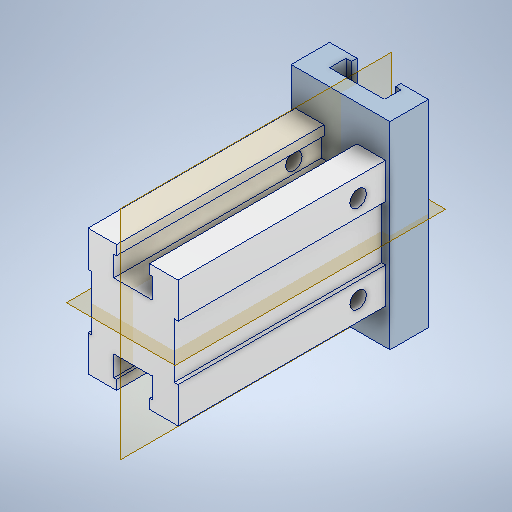
# Autodesk Inventor part: Cylinder
Saved by Autodesk Inventor 2025 (Build 290162000, 162)
## iProperties
Created: 2024-09-26
Part Number: Cylinder
Material: Aluminum 6061
Document SubType Name: Modeling
Designer: DMIADX
Density: 2.7 g/cm^3
Appearance: Aluminum - Flat
Author: DMIADX
Autodesk Inventor part; units mm, degrees
ref_plane "XY Plane" through (0, 0, 0) normal (0, 0, 1) x (1, 0, 0)
sketch "Sketch1" plane through (0, 0, 0) normal (0, 0, 1) x (1, 0, 0)
  line L0 (8.2, -11.5) -> (-8.2, -11.5)
  line L1 (-8.2, -11.5) -> (-8.2, 11.5)
  line L2 (-8.2, 11.5) -> (8.2, 11.5)
  line L3 (8.2, 11.5) -> (8.2, -11.5)
  line L4 (8.2, -11.5) -> (-8.2, 11.5) construction
  line L5 (-8.2, -11.5) -> (8.2, 11.5) construction
  line L6 (8.2, -5) -> (-8.2, -5)
  line L7 (-8.2, -5) -> (-8.2, 5)
  line L8 (-8.2, 5) -> (8.2, 5)
  line L9 (8.2, 5) -> (8.2, -5)
  line L10 (8.2, -5) -> (-8.2, 5) construction
  line L11 (-8.2, -5) -> (8.2, 5) construction
  line L12 (7.5, -5) -> (-7.5, -5)
  line L13 (-7.5, -5) -> (-7.5, 5)
  line L14 (-7.5, 5) -> (7.5, 5)
  line L15 (7.5, 5) -> (7.5, -5)
  line L16 (7.5, -5) -> (-7.5, 5) construction
  line L17 (-7.5, -5) -> (7.5, 5) construction
  line L18 (3, -11.5) -> (-3, -11.5)
  line L19 (-3, -11.5) -> (-3, 11.5)
  line L20 (-3, 11.5) -> (3, 11.5)
  line L21 (3, 11.5) -> (3, -11.5)
  line L22 (3, -11.5) -> (-3, 11.5) construction
  line L23 (-3, -11.5) -> (3, 11.5) construction
  line L24 (3.5, -9.75) -> (-3.5, -9.75)
  line L25 (-3.5, -9.75) -> (-3.5, 9.75)
  line L26 (-3.5, 9.75) -> (3.5, 9.75)
  line L27 (3.5, 9.75) -> (3.5, -9.75)
  line L28 (3.5, -9.75) -> (-3.5, 9.75) construction
  line L29 (-3.5, -9.75) -> (3.5, 9.75) construction
  line L30 (3.5, -6) -> (-3.5, -6)
  line L31 (-3.5, -6) -> (-3.5, 6)
  line L32 (-3.5, 6) -> (3.5, 6)
  line L33 (3.5, 6) -> (3.5, -6)
  line L34 (3.5, -6) -> (-3.5, 6) construction
  line L35 (-3.5, -6) -> (3.5, 6) construction
  point P0 (0, 0)
  point P1 (-3, -9.75)
  point P2 (3, -9.75)
  point P3 (3, 9.75)
  point P4 (-3, 9.75)
  dimension "d0" = 23
  dimension "d1" = 16.4
  dimension "d2" = 10
  dimension "d3" = 15
  dimension "d4" = 6
  dimension "d5" = 19.5
  dimension "d6" = 7
  dimension "d7" = 12
  constraints: 72 end point, 12 midpoint, 12 parallel, 6 horizontal, 6 perpendicular, 4 point on line
  measures "d0" distance of L0.end L1.end
  measures "d1" distance of L0.start L0.end
  measures "d2" distance of L12.end L13.end
  measures "d3" distance between parallel lines of L15 L13
  measures "d4" distance between parallel lines of L21 L19
  measures "d5" distance between parallel lines of L24 L26
  measures "d6" distance of L25.end L26.end
  measures "d7" distance between parallel lines of L30 L32
extrude "Extrusion1" add sketch "Sketch1" along normal blind 37.8 contours L0 L21 L24 L27 L6 L3 | L0 L1 L6 L25 L24 L19 | L8 L27 L26 L21 L2 L3 | L6 L27 L8 L15 | L30 L19 L6 L21 | L21 L6 L27 L30 | L6 L21 L8 L27 | L30 L25 L6 L19 | L6 L19 L8 L21 | L8 L21 L32 L27 | L1 L2 L19 L26 L25 L8 | L13 L8 L25 L6 | L6 L25 L8 L19 | L8 L19 L32 L21 | L8 L25 L32 L19
sketch "Sketch2" plane through (0, 0, 0) normal (1, 0, 0) x (0, 1, 0)
  circle A0 centre (-8, 5) radius 1.5
  circle A1 centre (8, 5) radius 1.5
  line L0 (-6, 0) -> (-6, 37.8) projected
  line L1 (6, 10) -> (-6, 10)
  line L2 (-6, 10) -> (-6, 0)
  line L3 (-6, 0) -> (6, 0)
  line L4 (6, 0) -> (6, 10)
  line L5 (6, 10) -> (-6, 0) construction
  line L6 (-6, 10) -> (6, 0) construction
  point P0 (0, 0)
  point P1 (0, 5)
  point P2 (-6, 10)
  dimension "d10" = 3
  dimension "d11" = 3
  dimension "d12" = 16
  dimension "d13" = 8
  dimension "d14" = 5
  dimension "d17" = 10
  constraints: 12 end point, 2 centre point, 2 midpoint, 2 parallel, 1 horizontal, 1 horizontal alignment, 1 perpendicular
  measures "d10" diameter of A0
  measures "d11" diameter of A1
  measures "d12" distance of A0.centre A1.centre
  measures "d13" horizontal distance of point (0, 0) A0.centre
  measures "d14" vertical distance of point (0, 0) A1.centre
  measures "d17" distance between parallel lines of L3 L1
extrude "Extrusion2" cut sketch "Sketch2" along normal through all both and the other way through all contours A0 | A1
sketch "Sketch3" plane through (0, 0, 0) normal (0, 0, -1) x (-1, 0, 0)
  line L0 (5, 18) -> (-5, 18)
  line L1 (-5, 18) -> (-5, -18)
  line L2 (-5, -18) -> (5, -18)
  line L3 (5, -18) -> (5, 18)
  line L4 (5, 18) -> (-5, -18) construction
  line L5 (-5, 18) -> (5, -18) construction
  line L6 (9, 18) -> (-9, 18)
  line L7 (-9, 18) -> (-9, -18)
  line L8 (-9, -18) -> (9, -18)
  line L9 (9, -18) -> (9, 18)
  line L10 (9, 18) -> (-9, -18) construction
  line L11 (-9, 18) -> (9, -18) construction
  line L12 (4, 18) -> (-4, 18)
  line L13 (-4, 18) -> (-4, -18)
  line L14 (-4, -18) -> (4, -18)
  line L15 (4, -18) -> (4, 18)
  line L16 (4, 18) -> (-4, -18) construction
  line L17 (-4, 18) -> (4, -18) construction
  point P0 (0, 0)
  point P1 (0, 18)
  point P2 (-5, 18)
  dimension "d20" = 10
  dimension "d21" = 18
  dimension "d22" = 36
  dimension "d23" = 36
  dimension "d24" = 8
  constraints: 36 end point, 7 midpoint, 6 parallel, 3 horizontal, 3 perpendicular, 1 point on line
  measures "d20" distance of L1.end L2.end
  measures "d21" distance of L7.end L8.end
  measures "d22" distance between parallel lines of L6 L8
  measures "d23" distance from line of point (0, 18) L2
  measures "d24" distance between parallel lines of L15 L13
extrude "Extrusion4" add sketch "Sketch3" along normal blind 7 contours L3 L2 L15 L0 | L6 L9 L8 L3 | L13 L2 L1 L0 | L1 L8 L7 L6
extrude "Extrusion5" cut sketch "Sketch3" along normal blind 6 contours L3 L2 L15 L0 | L13 L2 L1 L0
extrude "Extrusion6" add sketch "Sketch3" along normal blind 3 contours L3 L2 L15 L0 | L15 L2 L13 L0 | L13 L2 L1 L0
body "Solid1"
